Autodesk Inventor part; units mm, degrees
(part 2 of 2)
sketch "スケッチ4" plane through (0, 0, 0) normal (0, 0, 1) x (1, 0, 0)
  circle A0 centre (0, 0) radius 11.0288
  circle A1 centre (0, 0) radius 27.25
  circle A2 centre (0, 0) radius 22.25
  circle A3 centre (0, 0) radius 11.5288
  line L0 (-27.25, 0) -> (27.25, 0)
  line L1 (0, -27.25) -> (0, 27.25)
  line L2 (22.1994, 1.5) -> (11.2545, 2.5)
  line L3 (22.1994, -1.5) -> (11.2545, -2.5)
  line L4 (2.5, -11.2545) -> (1.5, -22.1994)
  line L5 (-2.5, -11.2545) -> (-1.5, -22.1994)
  line L6 (-22.1994, -1.5) -> (-11.2545, -2.5)
  line L7 (-11.2545, 2.5) -> (-22.1994, 1.5)
  line L8 (-1.5, 22.1994) -> (-2.5, 11.2545)
  line L9 (2.5, 11.2545) -> (1.5, 22.1994)
  point P0 (10.1524, 4.3085)
  point P1 (19.2887, 19.2486)
  dimension "d8" = 0.5
  dimension "d7" = 5
  dimension "d9" = 1.5
  dimension "d10" = 1.5
  dimension "d11" = 1.5
  dimension "d12" = 1.5
  dimension "d13" = 1.5
  dimension "d14" = 1.5
  dimension "d15" = 1.5
  dimension "d16" = 1.5
  dimension "d17" = 2.5
  dimension "d18" = 2.5
  dimension "d19" = 2.5
  dimension "d20" = 2.5
  dimension "d21" = 2.5
  dimension "d22" = 2.5
  dimension "d23" = 2.5
  dimension "d24" = 2.5
  constraints: 20 end point, 3 coincident, 3 point on circle, 2 midpoint, 1 centre point, 1 horizontal, 1 vertical, 23 other
  measures "d9" distance from line of L0 L3.start
  measures "d10" distance from line of L0 L2.start
  measures "d11" distance from line of L1 L4.end
  measures "d12" distance from line of L5.end L1
  measures "d13" distance from line of L0 L6.start
  measures "d14" distance from line of L0 L7.end
  measures "d15" distance from line of L1 L8.start
  measures "d16" distance from line of L1 L9.end
  measures "d17" distance from line of L0 L2.end
  measures "d18" distance from line of L3.end L0
  measures "d19" distance from line of L1 L4.start
  measures "d20" distance from line of L1 L5.start
  measures "d21" distance from line of L0 L6.end
  measures "d22" distance from line of L0 L7.start
  measures "d23" distance from line of L1 L8.end
  measures "d24" distance from line of L1 L9.start
extrude "押し出し4" cut sketch "スケッチ4" against normal through all contours A3 L9 A2 L2 | L3 A2 L4 A3 | A3 L7 A2 L8 | L5 A2 L6 A3
fillet "フィレット1" radius 4 16 edges at (1.5, 22.1994, -2) (-1.5, 22.1994, -2) (-2.5, 11.2545, -2) (2.5, 11.2545, -2) (11.2545, 2.5, -2) (22.1994, 1.5, -2) (22.1994, -1.5, -2) (11.2545, -2.5, -2) (1.5, -22.1994, -2) (2.5, -11.2545, -2) (-1.5, -22.1994, -2) (-2.5, -11.2545, -2) (-11.2545, -2.5, -2) (-22.1994, -1.5, -2) (-22.1994, 1.5, -2) (-11.2545, 2.5, -2)
sketch "スケッチ5" plane through (0, 0, 8) normal (0, 0, 1) x (1, 0, 0)
  arc A0 (-10.5551, -4.6371) -> (-4.6371, -10.5551) centre (0, 0) ccw projected
  arc A1 (-2.2625, -13.8534) -> (-4.6371, -10.5551) centre (-6.246, -14.2173) ccw projected
  line L0 (-2.2625, -13.8534) -> (-1.9858, -16.8822) projected
  arc A2 (-7.2775, -21.0262) -> (-1.9858, -16.8822) centre (-5.9692, -17.2462) ccw projected
  arc A3 (-21.0262, -7.2775) -> (-7.2775, -21.0262) centre (0, 0) ccw projected
  arc A4 (-16.8822, -1.9858) -> (-21.0262, -7.2775) centre (-17.2462, -5.9692) ccw projected
  line L1 (-16.8822, -1.9858) -> (-13.8534, -2.2625) projected
  arc A5 (-10.5551, -4.6371) -> (-13.8534, -2.2625) centre (-14.2173, -6.246) ccw projected
  line L2 (1.9858, -16.8822) -> (2.2625, -13.8534) projected
  arc A6 (4.6371, -10.5551) -> (2.2625, -13.8534) centre (6.246, -14.2173) ccw projected
  arc A7 (4.6371, -10.5551) -> (10.5551, -4.6371) centre (0, 0) ccw projected
  arc A8 (13.8534, -2.2625) -> (10.5551, -4.6371) centre (14.2173, -6.246) ccw projected
  line L3 (13.8534, -2.2625) -> (16.8822, -1.9858) projected
  arc A9 (21.0262, -7.2775) -> (16.8822, -1.9858) centre (17.2462, -5.9692) ccw projected
  arc A10 (7.2775, -21.0262) -> (21.0262, -7.2775) centre (0, 0) ccw projected
  arc A11 (1.9858, -16.8822) -> (7.2775, -21.0262) centre (5.9692, -17.2462) ccw projected
  line L4 (-1.9858, 16.8822) -> (-2.2625, 13.8534) projected
  arc A12 (-4.6371, 10.5551) -> (-2.2625, 13.8534) centre (-6.246, 14.2173) ccw projected
  arc A13 (-4.6371, 10.5551) -> (-10.5551, 4.6371) centre (0, 0) ccw projected
  arc A14 (-13.8534, 2.2625) -> (-10.5551, 4.6371) centre (-14.2173, 6.246) ccw projected
  line L5 (-13.8534, 2.2625) -> (-16.8822, 1.9858) projected
  arc A15 (-21.0262, 7.2775) -> (-16.8822, 1.9858) centre (-17.2462, 5.9692) ccw projected
  arc A16 (-7.2775, 21.0262) -> (-21.0262, 7.2775) centre (0, 0) ccw projected
  arc A17 (-1.9858, 16.8822) -> (-7.2775, 21.0262) centre (-5.9692, 17.2462) ccw projected
  arc A18 (21.0262, 7.2775) -> (7.2775, 21.0262) centre (0, 0) ccw projected
  arc A19 (16.8822, 1.9858) -> (21.0262, 7.2775) centre (17.2462, 5.9692) ccw projected
  line L6 (16.8822, 1.9858) -> (13.8534, 2.2625) projected
  arc A20 (10.5551, 4.6371) -> (13.8534, 2.2625) centre (14.2173, 6.246) ccw projected
  arc A21 (10.5551, 4.6371) -> (4.6371, 10.5551) centre (0, 0) ccw projected
  arc A22 (2.2625, 13.8534) -> (4.6371, 10.5551) centre (6.246, 14.2173) ccw projected
  line L7 (2.2625, 13.8534) -> (1.9858, 16.8822) projected
  arc A23 (7.2775, 21.0262) -> (1.9858, 16.8822) centre (5.9692, 17.2462) ccw projected
  arc A24 (-14.6125, 23.0008) -> (-14.9971, 23.3759) centre (-19.1364, 18.7478) ccw projected
  arc A25 (-14.9971, 23.3759) -> (-15.5935, 23.8634) centre (-20.7203, 16.9823) ccw projected
  arc A26 (-15.5935, 23.8634) -> (-16.4862, 24.4634) centre (-22.2157, 14.9751) ccw projected
  arc A27 (-16.4862, 24.4634) -> (-17.1295, 24.0173) centre (0, 0) ccw projected
  arc A28 (-17.1295, 24.0173) -> (-16.8828, 22.9783) centre (-6.2347, 26.0561) ccw projected
  arc A29 (-16.8828, 22.9783) -> (-16.6333, 22.2415) centre (-8.6388, 25.3594) ccw projected
  arc A30 (-16.6333, 22.2415) -> (-16.4168, 21.7498) centre (-10.8476, 24.4952) ccw projected
  arc A31 (-16.4168, 21.7498) -> (-17.0541, 21.2537) centre (0, 0) ccw projected
  arc A32 (-17.0541, 21.2537) -> (-17.4777, 21.5843) centre (-21.0827, 16.5289) ccw projected
  arc A33 (-17.4777, 21.5843) -> (-18.1241, 22.0031) centre (-22.4627, 14.5998) ccw projected
  arc A34 (-18.1241, 22.0031) -> (-19.0773, 22.5013) centre (-23.7282, 12.4403) ccw projected
  arc A35 (-19.0773, 22.5013) -> (-19.6677, 21.9871) centre (0, 0) ccw projected
  arc A36 (-19.6677, 21.9871) -> (-19.3081, 20.9816) centre (-9.0632, 25.2121) ccw projected
  arc A37 (-19.3081, 20.9816) -> (-18.9791, 20.2767) centre (-11.3761, 24.2551) ccw projected
  arc A38 (-18.9791, 20.2767) -> (-18.7098, 19.8118) centre (-13.4764, 23.1532) ccw projected
  arc A39 (-18.7098, 19.8118) -> (-19.2887, 19.2486) centre (0, 0) ccw projected
  arc A40 (-19.2887, 19.2486) -> (-19.746, 19.5306) centre (-22.773, 14.1093) ccw projected
  arc A41 (-19.746, 19.5306) -> (-20.4346, 19.8758) centre (-23.9325, 12.0401) ccw projected
  arc A42 (-20.4346, 19.8758) -> (-21.4368, 20.2661) centre (-24.9528, 9.7545) ccw projected
  arc A43 (-21.4368, 20.2661) -> (-21.9671, 19.69) centre (0, 0) ccw projected
  arc A44 (-21.9671, 19.69) -> (-21.4954, 18.7235) centre (-11.7818, 24.062) ccw projected
  arc A45 (-21.4954, 18.7235) -> (-21.0945, 18.0658) centre (-13.9753, 22.8564) ccw projected
  arc A46 (-21.0945, 18.0658) -> (-20.7757, 17.6333) centre (-15.9417, 21.5301) ccw projected
  arc A47 (-20.7757, 17.6333) -> (-21.2891, 17.0099) centre (0, 0) ccw projected
  arc A48 (-21.2891, 17.0099) -> (-21.7747, 17.2398) centre (-24.187, 11.5184) ccw projected
  arc A49 (-21.7747, 17.2398) -> (-22.4971, 17.5072) centre (-25.1117, 9.3343) ccw projected
  arc A50 (-22.4971, 17.5072) -> (-23.5361, 17.7848) centre (-25.8744, 6.9503) ccw projected
  arc A51 (-23.5361, 17.7848) -> (-23.9998, 17.154) centre (0, 0) ccw projected
  arc A52 (-23.9998, 17.154) -> (-23.4247, 16.2452) centre (-14.3573, 22.6199) ccw projected
  arc A53 (-23.4247, 16.2452) -> (-22.9538, 15.6355) centre (-16.4049, 21.1803) ccw projected
  arc A54 (-22.9538, 15.6355) -> (-22.5894, 15.2408) centre (-18.2134, 19.6457) ccw projected
  arc A55 (-22.5894, 15.2408) -> (-23.0312, 14.5646) centre (0, 0) ccw projected
  arc A56 (-23.0312, 14.5646) -> (-23.5391, 14.7398) centre (-25.3073, 8.7878) ccw projected
  arc A57 (-23.5391, 14.7398) -> (-24.294, 14.9276) centre (-25.9861, 6.5151) ccw projected
  arc A58 (-24.294, 14.9276) -> (-25.3498, 15.0877) centre (-26.4819, 4.0617) ccw projected
  arc A59 (-25.3498, 15.0877) -> (-25.7412, 14.4097) centre (0, 0) ccw projected
  arc A60 (-25.7412, 14.4097) -> (-25.0747, 13.5754) centre (-16.7585, 20.9032) ccw projected
  arc A61 (-25.0747, 13.5754) -> (-24.5345, 13.0155) centre (-18.6353, 19.2471) ccw projected
  arc A62 (-24.5345, 13.0155) -> (-24.1289, 12.6632) centre (-20.2641, 17.5229) ccw projected
  arc A63 (-24.1289, 12.6632) -> (-24.4936, 11.9426) centre (0, 0) ccw projected
  arc A64 (-24.4936, 11.9426) -> (-25.0177, 12.0608) centre (-26.1204, 5.9504) ccw projected
  arc A65 (-25.0177, 12.0608) -> (-25.7887, 12.1645) centre (-26.5451, 3.6169) ccw projected
  arc A66 (-25.7887, 12.1645) -> (-26.8557, 12.2075) centre (-26.768, 1.1238) ccw projected
  arc A67 (-26.8557, 12.2075) -> (-27.1702, 11.4905) centre (0, 0) ccw projected
  arc A68 (-27.1702, 11.4905) -> (-26.4159, 10.7346) centre (-18.9563, 18.9327) ccw projected
  arc A69 (-26.4159, 10.7346) -> (-25.8175, 10.2375) centre (-20.6396, 17.0802) ccw projected
  arc A70 (-25.8175, 10.2375) -> (-25.3755, 9.932) centre (-22.0687, 15.1873) ccw projected
  arc A71 (-25.3755, 9.932) -> (-25.6587, 9.1756) centre (0, 0) ccw projected
  arc A72 (-25.6587, 9.1756) -> (-26.1926, 9.2355) centre (-26.6165, 3.0408) ccw projected
  arc A73 (-26.1926, 9.2355) -> (-26.9703, 9.2537) centre (-26.7819, 0.6748) ccw projected
  arc A74 (-26.9703, 9.2537) -> (-28.0356, 9.179) centre (-26.7292, -1.8277) ccw projected
  arc A75 (-28.0356, 9.179) -> (-28.2693, 8.4318) centre (0, 0) ccw projected
  arc A76 (-28.2693, 8.4318) -> (-27.4364, 7.7635) centre (-20.924, 16.7325) ccw projected
  arc A77 (-27.4364, 7.7635) -> (-26.787, 7.3353) centre (-22.3933, 14.7061) ccw projected
  arc A78 (-26.787, 7.3353) -> (-26.3141, 7.0802) centre (-23.6055, 12.6674) ccw projected
  arc A79 (-26.3141, 7.0802) -> (-26.5124, 6.2973) centre (0, 0) ccw projected
  arc A80 (-26.5124, 6.2973) -> (-27.0496, 6.298) centre (-26.7894, 0.0943) ccw projected
  arc A81 (-27.0496, 6.298) -> (-27.8246, 6.2305) centre (-26.6936, -2.2756) ccw projected
  arc A82 (-27.8246, 6.2305) -> (-28.8752, 6.0392) centre (-26.3659, -4.757) ccw projected
  arc A83 (-28.8752, 6.0392) -> (-29.0253, 5.2708) centre (0, 0) ccw projected
  arc A84 (-29.0253, 5.2708) -> (-28.124, 4.6981) centre (-22.6377, 14.3291) ccw projected
  arc A85 (-28.124, 4.6981) -> (-27.4313, 4.344) centre (-23.8751, 12.1534) ccw projected
  arc A86 (-27.4313, 4.344) -> (-26.9333, 4.1425) centre (-24.8558, 9.9937) ccw projected
  arc A87 (-26.9333, 4.1425) -> (-27.0442, 3.3425) centre (0, 0) ccw projected
  arc A88 (-27.0442, 3.3425) -> (-27.5783, 3.2841) centre (-26.6372, -2.8533) ccw projected
  arc A89 (-27.5783, 3.2841) -> (-28.3412, 3.1318) centre (-26.2813, -5.1983) ccw projected
  arc A90 (-28.3412, 3.1318) -> (-29.3643, 2.826) centre (-25.6826, -7.6286) ccw projected
  arc A91 (-29.3643, 2.826) -> (-29.429, 2.0458) centre (0, 0) ccw projected
  arc A92 (-29.429, 2.0458) -> (-28.4631, 1.5727) centre (-24.0767, 11.7518) ccw projected
  arc A93 (-28.4631, 1.5727) -> (-27.7427, 1.2999) centre (-25.0672, 9.4531) ccw projected
  arc A94 (-27.7427, 1.2999) -> (-27.2255, 1.1544) centre (-25.8043, 7.1987) ccw projected
  arc A95 (-27.2255, 1.1544) -> (-27.2478, 0.3471) centre (0, 0) ccw projected
  arc A96 (-27.2478, 0.3471) -> (-27.7722, 0.2303) centre (-26.1617, -5.7663) ccw projected
  arc A97 (-27.7722, 0.2303) -> (-28.5137, -0.005) centre (-25.5499, -8.0579) ccw projected
  arc A98 (-28.5137, -0.005) -> (-29.497, -0.4215) centre (-24.6875, -10.4076) ccw projected
  arc A99 (-29.497, -0.4215) -> (-29.4754, -1.2041) centre (0, 0) ccw projected
  arc A100 (-29.4754, -1.2041) -> (-28.4706, -1.5658) centre (-25.2233, 9.0318) ccw projected
  arc A101 (-28.4706, -1.5658) -> (-27.7173, -1.7599) centre (-25.955, 6.6382) ccw projected
  arc A102 (-27.7173, -1.7599) -> (-27.1873, -1.8476) centre (-26.4396, 4.3163) ccw projected
  arc A103 (-27.1873, -1.8476) -> (-27.1206, -2.6525) centre (0, 0) ccw projected
  arc A104 (-27.1206, -2.6525) -> (-27.629, -2.8262) centre (-25.3685, -8.6093) ccw projected
  arc A105 (-27.629, -2.8262) -> (-28.3401, -3.1417) centre (-24.5084, -10.8197) ccw projected
  arc A106 (-28.3401, -3.1417) -> (-29.2716, -3.6638) centre (-23.3927, -13.0603) ccw projected
  arc A107 (-29.2716, -3.6638) -> (-29.1641, -4.4393) centre (0, 0) ccw projected
  arc A108 (-29.1641, -4.4393) -> (-28.1256, -4.6883) centre (-26.0638, 6.2023) ccw projected
  arc A109 (-28.1256, -4.6883) -> (-27.3555, -4.7983) centre (-26.5277, 3.7426) ccw projected
  arc A110 (-27.3555, -4.7983) -> (-26.819, -4.8272) centre (-26.754, 1.3816) ccw projected
  arc A111 (-26.819, -4.8272) -> (-26.6642, -5.6199) centre (0, 0) ccw projected
  arc A112 (-26.6642, -5.6199) -> (-27.1504, -5.8485) centre (-24.2675, -11.3478) ccw projected
  arc A113 (-27.1504, -5.8485) -> (-27.8224, -6.2403) centre (-23.1694, -13.4501) ccw projected
  arc A114 (-27.8224, -6.2403) -> (-28.6909, -6.8617) centre (-21.814, -15.5544) ccw projected
  arc A115 (-28.6909, -6.8617) -> (-28.4987, -7.6207) centre (0, 0) ccw projected
  arc A116 (-28.4987, -7.6207) -> (-27.4392, -7.7539) centre (-26.5879, 3.2974) ccw projected
  arc A117 (-27.4392, -7.7539) -> (-26.6616, -7.7786) centre (-26.7784, 0.8016) ccw projected
  arc A118 (-26.6616, -7.7786) -> (-26.1252, -7.7482) centre (-26.7436, -1.57) ccw projected
  arc A119 (-26.1252, -7.7482) -> (-25.8841, -8.519) centre (0, 0) ccw projected
  arc A120 (-25.8841, -8.519) -> (-26.3422, -8.7998) centre (-22.8719, -13.9485) ccw projected
  arc A121 (-26.3422, -8.7998) -> (-26.9671, -9.2631) centre (-21.5491, -15.9173) ccw projected
  arc A122 (-26.9671, -9.2631) -> (-27.7619, -9.9763) centre (-19.9705, -17.8597) ccw projected
  arc A123 (-27.7619, -9.9763) -> (-27.4874, -10.7095) centre (0, 0) ccw projected
  arc A124 (-27.4874, -10.7095) -> (-26.4196, -10.7253) centre (-26.7893, 0.3525) ccw projected
  arc A125 (-26.4196, -10.7253) -> (-25.6441, -10.6643) centre (-26.7041, -2.1491) ccw projected
  arc A126 (-25.6441, -10.6643) -> (-25.1143, -10.5752) centre (-26.4085, -4.5025) ccw projected
  arc A127 (-25.1143, -10.5752) -> (-24.7899, -11.3148) centre (0, 0) ccw projected
  arc A128 (-24.7899, -11.3148) -> (-25.2143, -11.6442) centre (-21.1986, -16.38) ccw projected
  arc A129 (-25.2143, -11.6442) -> (-25.7844, -12.1735) centre (-19.6673, -18.1913) ccw projected
  arc A130 (-25.7844, -12.1735) -> (-26.4959, -12.9698) centre (-17.8846, -19.9482) ccw projected
  arc A131 (-26.4959, -12.9698) -> (-26.1424, -13.6683) centre (0, 0) ccw projected
  arc A132 (-26.1424, -13.6683) -> (-25.0794, -13.5666) centre (-26.6655, -2.5967) ccw projected
  arc A133 (-25.0794, -13.5666) -> (-24.3153, -13.4207) centre (-26.3056, -5.0737) ccw projected
  arc A134 (-24.3153, -13.4207) -> (-23.7985, -13.2738) centre (-25.7529, -7.3803) ccw projected
  arc A135 (-23.7985, -13.2738) -> (-23.3947, -13.9732) centre (0, 0) ccw projected
  arc A136 (-23.3947, -13.9732) -> (-23.7803, -14.3473) centre (-19.268, -18.6126) ccw projected
  arc A137 (-23.7803, -14.3473) -> (-24.2887, -14.9361) centre (-17.5468, -20.2445) ccw projected
  arc A138 (-24.2887, -14.9361) -> (-24.9083, -15.8058) centre (-15.5815, -21.7946) ccw projected
  arc A139 (-24.9083, -15.8058) -> (-24.4801, -16.4613) centre (0, 0) ccw projected
  arc A140 (-24.4801, -16.4613) -> (-23.4347, -16.2432) centre (-26.218, -5.5144) ccw projected
  arc A141 (-23.4347, -16.2432) -> (-22.6913, -16.0141) centre (-25.5878, -7.9368) ccw projected
  arc A142 (-22.6913, -16.0141) -> (-22.1938, -15.8113) centre (-24.7848, -10.1685) ccw projected
  arc A143 (-22.1938, -15.8113) -> (-21.7155, -16.462) centre (0, 0) ccw projected
  arc A144 (-21.7155, -16.462) -> (-22.0576, -16.8763) centre (-17.1035, -20.6192) ccw projected
  arc A145 (-22.0576, -16.8763) -> (-22.4982, -17.5174) centre (-15.2132, -22.0519) ccw projected
  arc A146 (-22.4982, -17.5174) -> (-23.0184, -18.45) centre (-13.0894, -23.3764) ccw projected
  arc A147 (-23.0184, -18.45) -> (-22.5207, -19.0544) centre (0, 0) ccw projected
  arc A148 (-22.5207, -19.0544) -> (-21.5056, -18.7227) centre (-25.4522, -8.3651) ccw projected
  arc A149 (-21.5056, -18.7227) -> (-20.7919, -18.4131) centre (-24.5594, -10.7034) ccw projected
  arc A150 (-20.7919, -18.4131) -> (-20.3198, -18.1568) centre (-23.5157, -12.8333) ccw projected
  arc A151 (-20.3198, -18.1568) -> (-19.7728, -18.751) centre (0, 0) ccw projected
  arc A152 (-19.7728, -18.751) -> (-20.0672, -19.2004) centre (-14.7314, -22.3756) ccw projected
  arc A153 (-20.0672, -19.2004) -> (-20.4346, -19.8861) centre (-12.695, -23.5916) ccw projected
  arc A154 (-20.4346, -19.8861) -> (-20.849, -20.8703) centre (-10.4383, -24.6745) ccw projected
  arc A155 (-20.849, -20.8703) -> (-20.2879, -21.4162) centre (0, 0) ccw projected
  arc A156 (-20.2879, -21.4162) -> (-19.3155, -20.9748) centre (-24.3775, -11.1143) ccw projected
  arc A157 (-19.3155, -20.9748) -> (-18.6401, -20.5887) centre (-23.2328, -13.3402) ccw projected
  arc A158 (-18.6401, -20.5887) -> (-18.1991, -20.2819) centre (-21.9612, -15.3424) ccw projected
  arc A159 (-18.1991, -20.2819) -> (-17.59, -20.8124) centre (0, 0) ccw projected
  arc A160 (-17.59, -20.8124) -> (-17.8332, -21.2914) centre (-12.1805, -23.8604) ccw projected
  arc A161 (-17.8332, -21.2914) -> (-18.123, -22.0133) centre (-10.0227, -24.845) ccw projected
  arc A162 (-18.123, -22.0133) -> (-18.4266, -23.0372) centre (-7.6606, -25.6731) ccw projected
  arc A163 (-18.4266, -23.0372) -> (-17.8088, -23.518) centre (0, 0) ccw projected
  arc A164 (-17.8088, -23.518) -> (-16.8908, -22.9724) centre (-23.0069, -13.7285) ccw projected
  arc A165 (-16.8908, -22.9724) -> (-16.2621, -22.5143) centre (-21.6243, -15.8151) ccw projected
  arc A166 (-16.2621, -22.5143) -> (-15.8574, -22.1609) centre (-20.1401, -17.6652) ccw projected
  arc A167 (-15.8574, -22.1609) -> (-15.1937, -22.6211) centre (0, 0) ccw projected
  arc A168 (-15.1937, -22.6211) -> (-15.3828, -23.124) centre (-9.4817, -25.0555) ccw projected
  arc A169 (-15.3828, -23.124) -> (-15.5913, -23.8734) centre (-7.2287, -25.7968) ccw projected
  arc A170 (-15.5913, -23.8734) -> (-15.7805, -24.9244) centre (-4.7899, -26.36) ccw projected
  arc A171 (-15.7805, -24.9244) -> (-15.1135, -25.3344) centre (0, 0) ccw projected
  arc A172 (-15.1135, -25.3344) -> (-14.2612, -24.6911) centre (-21.357, -16.1762) ccw projected
  arc A173 (-14.2612, -24.6911) -> (-13.6866, -24.1666) centre (-19.7533, -18.0979) ccw projected
  arc A174 (-13.6866, -24.1666) -> (-13.3233, -23.7708) centre (-18.0746, -19.7735) ccw projected
  arc A175 (-13.3233, -23.7708) -> (-12.613, -24.1552) centre (0, 0) ccw projected
  arc A176 (-12.613, -24.1552) -> (-12.7456, -24.6759) centre (-6.6679, -25.9465) ccw projected
  arc A177 (-12.7456, -24.6759) -> (-12.8704, -25.4437) centre (-4.347, -26.4354) ccw projected
  arc A178 (-12.8704, -25.4437) -> (-12.9428, -26.5091) centre (-1.861, -26.7269) ccw projected
  arc A179 (-12.9428, -26.5091) -> (-12.2348, -26.8433) centre (0, 0) ccw projected
  arc A180 (-12.2348, -26.8433) -> (-11.4584, -26.1101) centre (-19.4479, -18.4274) ccw projected
  arc A181 (-11.4584, -26.1101) -> (-10.945, -25.5256) centre (-17.6425, -20.1611) ccw projected
  arc A182 (-10.945, -25.5256) -> (-10.6274, -25.0922) centre (-15.7896, -21.6419) ccw projected
  arc A183 (-10.6274, -25.0922) -> (-9.8792, -25.3962) centre (0, 0) ccw projected
  arc A184 (-9.8792, -25.3962) -> (-9.9537, -25.9282) centre (-3.7731, -26.5226) ccw projected
  arc A185 (-9.9537, -25.9282) -> (-9.9933, -26.7051) centre (-1.4125, -26.7532) ccw projected
  arc A186 (-9.9933, -26.7051) -> (-9.948, -27.772) centre (1.0905, -26.7694) ccw projected
  arc A187 (-9.948, -27.772) -> (-9.2075, -28.0263) centre (0, 0) ccw projected
  arc A188 (-9.2075, -28.0263) -> (-8.5165, -27.2121) centre (-17.3027, -20.455) ccw projected
  arc A189 (-8.5165, -27.2121) -> (-8.0706, -26.5747) centre (-15.3175, -21.9796) ccw projected
  arc A190 (-8.0706, -26.5747) -> (-7.8026, -26.109) centre (-13.313, -23.2475) ccw projected
  arc A191 (-7.8026, -26.109) -> (-7.0254, -26.3288) centre (0, 0) ccw projected
  arc A192 (-7.0254, -26.3288) -> (-7.041, -26.8658) centre (-0.8325, -26.7767) ccw projected
  arc A193 (-7.041, -26.8658) -> (-6.9957, -27.6348) centre (1.5392, -26.7462) ccw projected
  arc A194 (-6.9957, -27.6348) -> (-6.8325, -28.6979) centre (4.0287, -26.487) ccw projected
  arc A195 (-6.8325, -28.6979) -> (-6.0685, -28.8691) centre (0, 0) ccw projected
  arc A196 (-6.0685, -28.8691) -> (-5.4713, -27.9838) centre (-14.9474, -22.2343) ccw projected
  arc A197 (-5.4713, -27.9838) -> (-5.0982, -27.3012) centre (-12.8066, -23.5312) ccw projected
  arc A198 (-5.0982, -27.3012) -> (-4.883, -26.8089) centre (-10.6748, -24.571) ccw projected
  arc A199 (-4.883, -26.8089) -> (-4.0864, -26.9419) centre (0, 0) ccw projected
  arc A200 (-4.0864, -26.9419) -> (-4.0428, -27.4773) centre (2.1182, -26.7057) ccw projected
  arc A201 (-4.0428, -27.4773) -> (-3.9115, -28.2441) centre (4.4721, -26.4145) ccw projected
  arc A202 (-3.9115, -28.2441) -> (-3.634, -29.2753) centre (6.9181, -25.883) ccw projected
  arc A203 (-3.634, -29.2753) -> (-2.8559, -29.3614) centre (0, 0) ccw projected
  arc A204 (-2.8559, -29.3614) -> (-2.3596, -28.4159) centre (-12.4108, -23.7437) ccw projected
  arc A205 (-2.3596, -28.4159) -> (-2.0639, -27.6964) centre (-10.1402, -24.7972) ccw projected
  arc A206 (-2.0639, -27.6964) -> (-1.9042, -27.1834) centre (-7.907, -25.5961) ccw projected
  arc A207 (-1.9042, -27.1834) -> (-1.0978, -27.2279) centre (0, 0) ccw projected
  arc A208 (-1.0978, -27.2279) -> (-0.9955, -27.7553) centre (5.0432, -26.3106) ccw projected
  arc A209 (-0.9955, -27.7553) -> (-0.7807, -28.503) centre (7.3508, -25.7622) ccw projected
  arc A210 (-0.7807, -28.503) -> (-0.3915, -29.4974) centre (9.7234, -24.9649) ccw projected
  arc A211 (-0.3915, -29.4974) -> (0.3915, -29.4974) centre (0, 0) ccw projected
  arc A212 (0.3915, -29.4974) -> (0.7807, -28.503) centre (-9.7234, -24.9649) ccw projected
  arc A213 (0.7807, -28.503) -> (0.9955, -27.7553) centre (-7.3508, -25.7622) ccw projected
  arc A214 (0.9955, -27.7553) -> (1.0978, -27.2279) centre (-5.0432, -26.3106) ccw projected
  arc A215 (1.0978, -27.2279) -> (1.9042, -27.1834) centre (0, 0) ccw projected
  arc A216 (1.9042, -27.1834) -> (2.0639, -27.6964) centre (7.907, -25.5961) ccw projected
  arc A217 (2.0639, -27.6964) -> (2.3596, -28.4159) centre (10.1402, -24.7972) ccw projected
  arc A218 (2.3596, -28.4159) -> (2.8559, -29.3614) centre (12.4108, -23.7437) ccw projected
  arc A219 (2.8559, -29.3614) -> (3.634, -29.2753) centre (0, 0) ccw projected
  arc A220 (3.634, -29.2753) -> (3.9115, -28.2441) centre (-6.9181, -25.883) ccw projected
  arc A221 (3.9115, -28.2441) -> (4.0428, -27.4773) centre (-4.4721, -26.4145) ccw projected
  arc A222 (4.0428, -27.4773) -> (4.0864, -26.9419) centre (-2.1182, -26.7057) ccw projected
  arc A223 (4.0864, -26.9419) -> (4.883, -26.8089) centre (0, 0) ccw projected
  arc A224 (4.883, -26.8089) -> (5.0982, -27.3012) centre (10.6748, -24.571) ccw projected
  arc A225 (5.0982, -27.3012) -> (5.4713, -27.9838) centre (12.8066, -23.5312) ccw projected
  arc A226 (5.4713, -27.9838) -> (6.0685, -28.8691) centre (14.9474, -22.2343) ccw projected
  arc A227 (6.0685, -28.8691) -> (6.8325, -28.6979) centre (0, 0) ccw projected
  arc A228 (6.8325, -28.6979) -> (6.9949, -27.6424) centre (-4.0287, -26.487) ccw projected
  arc A229 (6.9949, -27.6424) -> (7.041, -26.8658) centre (-1.5392, -26.7462) ccw projected
  arc A230 (7.041, -26.8658) -> (7.0254, -26.3288) centre (0.8325, -26.7767) ccw projected
  arc A231 (7.0254, -26.3288) -> (7.8026, -26.109) centre (0, 0) ccw projected
  arc A232 (7.8026, -26.109) -> (8.0706, -26.5747) centre (13.313, -23.2475) ccw projected
  arc A233 (8.0706, -26.5747) -> (8.5165, -27.2121) centre (15.3175, -21.9796) ccw projected
  arc A234 (8.5165, -27.2121) -> (9.2075, -28.0263) centre (17.3027, -20.455) ccw projected
  arc A235 (9.2075, -28.0263) -> (9.948, -27.772) centre (0, 0) ccw projected
  arc A236 (9.948, -27.772) -> (9.9933, -26.7051) centre (-1.0905, -26.7694) ccw projected
  arc A237 (9.9933, -26.7051) -> (9.9537, -25.9282) centre (1.4125, -26.7532) ccw projected
  arc A238 (9.9537, -25.9282) -> (9.8792, -25.3962) centre (3.7731, -26.5226) ccw projected
  arc A239 (9.8792, -25.3962) -> (10.6274, -25.0922) centre (0, 0) ccw projected
  arc A240 (10.6274, -25.0922) -> (10.945, -25.5256) centre (15.7896, -21.6419) ccw projected
  arc A241 (10.945, -25.5256) -> (11.4584, -26.1101) centre (17.6425, -20.1611) ccw projected
  arc A242 (11.4584, -26.1101) -> (12.2348, -26.8433) centre (19.4479, -18.4274) ccw projected
  arc A243 (12.2348, -26.8433) -> (12.9428, -26.5091) centre (0, 0) ccw projected
  arc A244 (12.9428, -26.5091) -> (12.8704, -25.4437) centre (1.861, -26.7269) ccw projected
  arc A245 (12.8704, -25.4437) -> (12.7456, -24.6759) centre (4.347, -26.4354) ccw projected
  arc A246 (12.7456, -24.6759) -> (12.613, -24.1552) centre (6.6679, -25.9465) ccw projected
  arc A247 (12.613, -24.1552) -> (13.3233, -23.7708) centre (0, 0) ccw projected
  arc A248 (13.3233, -23.7708) -> (13.6866, -24.1666) centre (18.0746, -19.7735) ccw projected
  arc A249 (13.6866, -24.1666) -> (14.2612, -24.6911) centre (19.7533, -18.0979) ccw projected
  arc A250 (14.2612, -24.6911) -> (15.1135, -25.3344) centre (21.357, -16.1762) ccw projected
  arc A251 (15.1135, -25.3344) -> (15.7805, -24.9244) centre (0, 0) ccw projected
  arc A252 (15.7805, -24.9244) -> (15.5913, -23.8734) centre (4.7899, -26.36) ccw projected
  arc A253 (15.5913, -23.8734) -> (15.3828, -23.124) centre (7.2287, -25.7968) ccw projected
  arc A254 (15.3828, -23.124) -> (15.1937, -22.6211) centre (9.4817, -25.0555) ccw projected
  arc A255 (15.1937, -22.6211) -> (15.8574, -22.1609) centre (0, 0) ccw projected
  arc A256 (15.8574, -22.1609) -> (16.2621, -22.5143) centre (20.1401, -17.6652) ccw projected
  arc A257 (16.2621, -22.5143) -> (16.8908, -22.9724) centre (21.6243, -15.8151) ccw projected
  arc A258 (16.8908, -22.9724) -> (17.8088, -23.518) centre (23.0069, -13.7285) ccw projected
  arc A259 (17.8088, -23.518) -> (18.4266, -23.0372) centre (0, 0) ccw projected
  arc A260 (18.4266, -23.0372) -> (18.123, -22.0134) centre (7.6606, -25.6731) ccw projected
  arc A261 (18.123, -22.0134) -> (17.8332, -21.2914) centre (10.0227, -24.845) ccw projected
  arc A262 (17.8332, -21.2914) -> (17.59, -20.8124) centre (12.1805, -23.8604) ccw projected
  arc A263 (17.59, -20.8124) -> (18.1991, -20.2819) centre (0, 0) ccw projected
  arc A264 (18.1991, -20.2819) -> (18.6401, -20.5887) centre (21.9612, -15.3424) ccw projected
  arc A265 (18.6401, -20.5887) -> (19.3155, -20.9748) centre (23.2328, -13.3402) ccw projected
  arc A266 (19.3155, -20.9748) -> (20.2879, -21.4162) centre (24.3775, -11.1143) ccw projected
  arc A267 (20.2879, -21.4162) -> (20.849, -20.8703) centre (0, 0) ccw projected
  arc A268 (20.849, -20.8703) -> (20.4313, -19.8792) centre (10.4383, -24.6745) ccw projected
  arc A269 (20.4313, -19.8792) -> (20.0672, -19.2004) centre (12.695, -23.5916) ccw projected
  arc A270 (20.0672, -19.2004) -> (19.7728, -18.751) centre (14.7314, -22.3756) ccw projected
  arc A271 (19.7728, -18.751) -> (20.3198, -18.1568) centre (0, 0) ccw projected
  arc A272 (20.3198, -18.1568) -> (20.7919, -18.4131) centre (23.5157, -12.8333) ccw projected
  arc A273 (20.7919, -18.4131) -> (21.5056, -18.7227) centre (24.5594, -10.7034) ccw projected
  arc A274 (21.5056, -18.7227) -> (22.5207, -19.0544) centre (25.4522, -8.3651) ccw projected
  arc A275 (22.5207, -19.0544) -> (23.0184, -18.45) centre (0, 0) ccw projected
  arc A276 (23.0184, -18.45) -> (22.4982, -17.5174) centre (13.0894, -23.3764) ccw projected
  arc A277 (22.4982, -17.5174) -> (22.0576, -16.8763) centre (15.2132, -22.0519) ccw projected
  arc A278 (22.0576, -16.8763) -> (21.7155, -16.462) centre (17.1035, -20.6192) ccw projected
  arc A279 (21.7155, -16.462) -> (22.1938, -15.8113) centre (0, 0) ccw projected
  arc A280 (22.1938, -15.8113) -> (22.6913, -16.0141) centre (24.7848, -10.1685) ccw projected
  arc A281 (22.6913, -16.0141) -> (23.4347, -16.2432) centre (25.5878, -7.9368) ccw projected
  arc A282 (23.4347, -16.2432) -> (24.4801, -16.4613) centre (26.218, -5.5144) ccw projected
  arc A283 (24.4801, -16.4613) -> (24.9083, -15.8058) centre (0, 0) ccw projected
  arc A284 (24.9083, -15.8058) -> (24.2887, -14.9361) centre (15.5815, -21.7946) ccw projected
  arc A285 (24.2887, -14.9361) -> (23.7803, -14.3473) centre (17.5468, -20.2445) ccw projected
  arc A286 (23.7803, -14.3473) -> (23.3947, -13.9732) centre (19.268, -18.6126) ccw projected
  arc A287 (23.3947, -13.9732) -> (23.7985, -13.2738) centre (0, 0) ccw projected
  arc A288 (23.7985, -13.2738) -> (24.3153, -13.4207) centre (25.7529, -7.3803) ccw projected
  arc A289 (24.3153, -13.4207) -> (25.0794, -13.5666) centre (26.3056, -5.0737) ccw projected
  arc A290 (25.0794, -13.5666) -> (26.1424, -13.6683) centre (26.6655, -2.5967) ccw projected
  arc A291 (26.1424, -13.6683) -> (26.4959, -12.9698) centre (0, 0) ccw projected
  arc A292 (26.4959, -12.9698) -> (25.7844, -12.1735) centre (17.8846, -19.9482) ccw projected
  arc A293 (25.7844, -12.1735) -> (25.2143, -11.6442) centre (19.6673, -18.1913) ccw projected
  arc A294 (25.2143, -11.6442) -> (24.7899, -11.3148) centre (21.1986, -16.38) ccw projected
  arc A295 (24.7899, -11.3148) -> (25.1143, -10.5752) centre (0, 0) ccw projected
  arc A296 (25.1143, -10.5752) -> (25.6441, -10.6643) centre (26.4085, -4.5025) ccw projected
  arc A297 (25.6441, -10.6643) -> (26.4196, -10.7253) centre (26.7041, -2.1491) ccw projected
  arc A298 (26.4196, -10.7253) -> (27.4874, -10.7095) centre (26.7893, 0.3525) ccw projected
  arc A299 (27.4874, -10.7095) -> (27.7619, -9.9763) centre (0, 0) ccw projected
  arc A300 (27.7619, -9.9763) -> (26.9671, -9.2631) centre (19.9705, -17.8597) ccw projected
  arc A301 (26.9671, -9.2631) -> (26.3422, -8.7998) centre (21.5491, -15.9173) ccw projected
  arc A302 (26.3422, -8.7998) -> (25.8841, -8.519) centre (22.8719, -13.9485) ccw projected
  arc A303 (25.8841, -8.519) -> (26.1252, -7.7482) centre (0, 0) ccw projected
  arc A304 (26.1252, -7.7482) -> (26.6616, -7.7786) centre (26.7436, -1.57) ccw projected
  arc A305 (26.6616, -7.7786) -> (27.4392, -7.7539) centre (26.7784, 0.8016) ccw projected
  arc A306 (27.4392, -7.7539) -> (28.4987, -7.6207) centre (26.5879, 3.2974) ccw projected
  arc A307 (28.4987, -7.6207) -> (28.6909, -6.8617) centre (0, 0) ccw projected
  arc A308 (28.6909, -6.8617) -> (27.8224, -6.2403) centre (21.814, -15.5544) ccw projected
  arc A309 (27.8224, -6.2403) -> (27.1504, -5.8485) centre (23.1694, -13.4501) ccw projected
  arc A310 (27.1504, -5.8485) -> (26.6642, -5.6199) centre (24.2675, -11.3478) ccw projected
  arc A311 (26.6642, -5.6199) -> (26.819, -4.8272) centre (0, 0) ccw projected
  arc A312 (26.819, -4.8272) -> (27.3555, -4.7983) centre (26.754, 1.3816) ccw projected
  arc A313 (27.3555, -4.7983) -> (28.1256, -4.6883) centre (26.5277, 3.7426) ccw projected
  arc A314 (28.1256, -4.6883) -> (29.1641, -4.4393) centre (26.0638, 6.2023) ccw projected
  arc A315 (29.1641, -4.4393) -> (29.2716, -3.6638) centre (0, 0) ccw projected
  arc A316 (29.2716, -3.6638) -> (28.3332, -3.1383) centre (23.3927, -13.0603) ccw projected
  arc A317 (28.3332, -3.1383) -> (27.629, -2.8262) centre (24.5084, -10.8197) ccw projected
  arc A318 (27.629, -2.8262) -> (27.1206, -2.6525) centre (25.3685, -8.6093) ccw projected
  arc A319 (27.1206, -2.6525) -> (27.1873, -1.8476) centre (0, 0) ccw projected
  arc A320 (27.1873, -1.8476) -> (27.7173, -1.7599) centre (26.4396, 4.3163) ccw projected
  arc A321 (27.7173, -1.7599) -> (28.4707, -1.5658) centre (25.955, 6.6382) ccw projected
  arc A322 (28.4707, -1.5658) -> (29.4754, -1.2041) centre (25.2233, 9.0318) ccw projected
  arc A323 (29.4754, -1.2041) -> (29.497, -0.4215) centre (0, 0) ccw projected
  arc A324 (29.497, -0.4215) -> (28.5065, -0.0023) centre (24.6875, -10.4076) ccw projected
  arc A325 (28.5065, -0.0023) -> (27.7722, 0.2303) centre (25.5499, -8.0579) ccw projected
  arc A326 (27.7722, 0.2303) -> (27.2478, 0.3471) centre (26.1617, -5.7663) ccw projected
  arc A327 (27.2478, 0.3471) -> (27.2255, 1.1544) centre (0, 0) ccw projected
  arc A328 (27.2255, 1.1544) -> (27.7427, 1.2999) centre (25.8043, 7.1987) ccw projected
  arc A329 (27.7427, 1.2999) -> (28.4701, 1.5757) centre (25.0672, 9.4531) ccw projected
  arc A330 (28.4701, 1.5757) -> (29.429, 2.0458) centre (24.0767, 11.7518) ccw projected
  arc A331 (29.429, 2.0458) -> (29.3643, 2.826) centre (0, 0) ccw projected
  arc A332 (29.3643, 2.826) -> (28.3412, 3.1318) centre (25.6826, -7.6286) ccw projected
  arc A333 (28.3412, 3.1318) -> (27.5783, 3.2841) centre (26.2813, -5.1983) ccw projected
  arc A334 (27.5783, 3.2841) -> (27.0442, 3.3425) centre (26.6372, -2.8533) ccw projected
  arc A335 (27.0442, 3.3425) -> (26.9333, 4.1425) centre (0, 0) ccw projected
  arc A336 (26.9333, 4.1425) -> (27.4313, 4.344) centre (24.8558, 9.9937) ccw projected
  arc A337 (27.4313, 4.344) -> (28.124, 4.6981) centre (23.8751, 12.1534) ccw projected
  arc A338 (28.124, 4.6981) -> (29.0253, 5.2708) centre (22.6377, 14.3291) ccw projected
  arc A339 (29.0253, 5.2708) -> (28.8752, 6.0392) centre (0, 0) ccw projected
  arc A340 (28.8752, 6.0392) -> (27.8246, 6.2305) centre (26.3659, -4.757) ccw projected
  arc A341 (27.8246, 6.2305) -> (27.0496, 6.298) centre (26.6936, -2.2756) ccw projected
  arc A342 (27.0496, 6.298) -> (26.5124, 6.2973) centre (26.7894, 0.0943) ccw projected
  arc A343 (26.5124, 6.2973) -> (26.3141, 7.0802) centre (0, 0) ccw projected
  arc A344 (26.3141, 7.0802) -> (26.787, 7.3353) centre (23.6055, 12.6674) ccw projected
  arc A345 (26.787, 7.3353) -> (27.4364, 7.7635) centre (22.3933, 14.7061) ccw projected
  arc A346 (27.4364, 7.7635) -> (28.2693, 8.4318) centre (20.924, 16.7325) ccw projected
  arc A347 (28.2693, 8.4318) -> (28.0356, 9.179) centre (0, 0) ccw projected
  arc A348 (28.0356, 9.179) -> (26.9703, 9.2537) centre (26.7292, -1.8277) ccw projected
  arc A349 (26.9703, 9.2537) -> (26.1926, 9.2355) centre (26.7819, 0.6748) ccw projected
  arc A350 (26.1926, 9.2355) -> (25.6587, 9.1756) centre (26.6165, 3.0408) ccw projected
  arc A351 (25.6587, 9.1756) -> (25.3755, 9.932) centre (0, 0) ccw projected
  arc A352 (25.3755, 9.932) -> (25.8175, 10.2375) centre (22.0687, 15.1873) ccw projected
  arc A353 (25.8175, 10.2375) -> (26.4159, 10.7346) centre (20.6396, 17.0802) ccw projected
  arc A354 (26.4159, 10.7346) -> (27.1702, 11.4905) centre (18.9563, 18.9327) ccw projected
  arc A355 (27.1702, 11.4905) -> (26.8557, 12.2075) centre (0, 0) ccw projected
  arc A356 (26.8557, 12.2075) -> (25.7887, 12.1645) centre (26.768, 1.1238) ccw projected
  arc A357 (25.7887, 12.1645) -> (25.0177, 12.0608) centre (26.5451, 3.6169) ccw projected
  arc A358 (25.0177, 12.0608) -> (24.4936, 11.9426) centre (26.1204, 5.9504) ccw projected
  arc A359 (24.4936, 11.9426) -> (24.1289, 12.6632) centre (0, 0) ccw projected
  arc A360 (24.1289, 12.6632) -> (24.5345, 13.0155) centre (20.2641, 17.5229) ccw projected
  arc A361 (24.5345, 13.0155) -> (25.0747, 13.5754) centre (18.6353, 19.2471) ccw projected
  arc A362 (25.0747, 13.5754) -> (25.7412, 14.4097) centre (16.7585, 20.9032) ccw projected
  arc A363 (25.7412, 14.4097) -> (25.3498, 15.0877) centre (0, 0) ccw projected
  arc A364 (25.3498, 15.0877) -> (24.294, 14.9276) centre (26.4819, 4.0617) ccw projected
  arc A365 (24.294, 14.9276) -> (23.5391, 14.7398) centre (25.9861, 6.5151) ccw projected
  arc A366 (23.5391, 14.7398) -> (23.0312, 14.5646) centre (25.3073, 8.7878) ccw projected
  arc A367 (23.0312, 14.5646) -> (22.5894, 15.2408) centre (0, 0) ccw projected
  arc A368 (22.5894, 15.2408) -> (22.9538, 15.6355) centre (18.2134, 19.6457) ccw projected
  arc A369 (22.9538, 15.6355) -> (23.4291, 16.2514) centre (16.4049, 21.1803) ccw projected
  arc A370 (23.4291, 16.2514) -> (23.9998, 17.154) centre (14.3573, 22.6199) ccw projected
  arc A371 (23.9998, 17.154) -> (23.5361, 17.7848) centre (0, 0) ccw projected
  arc A372 (23.5361, 17.7848) -> (22.5044, 17.5095) centre (25.8744, 6.9503) ccw projected
  arc A373 (22.5044, 17.5095) -> (21.7747, 17.2398) centre (25.1117, 9.3343) ccw projected
  arc A374 (21.7747, 17.2398) -> (21.2891, 17.0099) centre (24.187, 11.5184) ccw projected
  arc A375 (21.2891, 17.0099) -> (20.7757, 17.6333) centre (0, 0) ccw projected
  arc A376 (20.7757, 17.6333) -> (21.0945, 18.0658) centre (15.9417, 21.5301) ccw projected
  arc A377 (21.0945, 18.0658) -> (21.4991, 18.7302) centre (13.9753, 22.8564) ccw projected
  arc A378 (21.4991, 18.7302) -> (21.9671, 19.69) centre (11.7818, 24.062) ccw projected
  arc A379 (21.9671, 19.69) -> (21.4368, 20.2661) centre (0, 0) ccw projected
  arc A380 (21.4368, 20.2661) -> (20.4416, 19.8789) centre (24.9528, 9.7545) ccw projected
  arc A381 (20.4416, 19.8789) -> (19.746, 19.5306) centre (23.9325, 12.0401) ccw projected
  arc A382 (19.746, 19.5306) -> (19.2887, 19.2486) centre (22.773, 14.1093) ccw projected
  arc A383 (19.2887, 19.2486) -> (18.7098, 19.8118) centre (0, 0) ccw projected
  arc A384 (18.7098, 19.8118) -> (18.9791, 20.2767) centre (13.4764, 23.1532) ccw projected
  arc A385 (18.9791, 20.2767) -> (19.3081, 20.9816) centre (11.3761, 24.2551) ccw projected
  arc A386 (19.3081, 20.9816) -> (19.6677, 21.9871) centre (9.0632, 25.2121) ccw projected
  arc A387 (19.6677, 21.9871) -> (19.0773, 22.5013) centre (0, 0) ccw projected
  arc A388 (19.0773, 22.5013) -> (18.1307, 22.007) centre (23.7282, 12.4403) ccw projected
  arc A389 (18.1307, 22.007) -> (17.4777, 21.5843) centre (22.4627, 14.5998) ccw projected
  arc A390 (17.4777, 21.5843) -> (17.0541, 21.2537) centre (21.0827, 16.5289) ccw projected
  arc A391 (17.0541, 21.2537) -> (16.4168, 21.7498) centre (0, 0) ccw projected
  arc A392 (16.4168, 21.7498) -> (16.6333, 22.2415) centre (10.8476, 24.4952) ccw projected
  arc A393 (16.6333, 22.2415) -> (16.8828, 22.9783) centre (8.6388, 25.3594) ccw projected
  arc A394 (16.8828, 22.9783) -> (17.1295, 24.0173) centre (6.2347, 26.0561) ccw projected
  arc A395 (17.1295, 24.0173) -> (16.4862, 24.4634) centre (0, 0) ccw projected
  arc A396 (16.4862, 24.4634) -> (15.5997, 23.868) centre (22.2157, 14.9751) ccw projected
  arc A397 (15.5997, 23.868) -> (14.9971, 23.3759) centre (20.7203, 16.9823) ccw projected
  arc A398 (14.9971, 23.3759) -> (14.6125, 23.0008) centre (19.1364, 18.7478) ccw projected
  arc A399 (14.6125, 23.0008) -> (13.9245, 23.4237) centre (0, 0) ccw projected
  arc A400 (13.9245, 23.4237) -> (14.0856, 23.9363) centre (8.0871, 25.5398) ccw projected
  arc A401 (14.0856, 23.9363) -> (14.2525, 24.6961) centre (5.7966, 26.1558) ccw projected
  arc A402 (14.2525, 24.6961) -> (14.3835, 25.7559) centre (3.3305, 26.5838) ccw projected
  arc A403 (14.3835, 25.7559) -> (13.6949, 26.1285) centre (0, 0) ccw projected
  arc A404 (13.6949, 26.1285) -> (12.8793, 25.4392) centre (20.4335, 17.3281) ccw projected
  arc A405 (12.8793, 25.4392) -> (12.3346, 24.8839) centre (18.7263, 19.1586) ccw projected
  arc A406 (12.3346, 24.8839) -> (11.9936, 24.4687) centre (16.9579, 20.7392) ccw projected
  arc A407 (11.9936, 24.4687) -> (11.2632, 24.8134) centre (0, 0) ccw projected
  arc A408 (11.2632, 24.8134) -> (11.3669, 25.3405) centre (5.2284, 26.2744) ccw projected
  arc A409 (11.3669, 25.3405) -> (11.4492, 26.1141) centre (2.8841, 26.6347) ccw projected
  arc A410 (11.4492, 26.1141) -> (11.4628, 27.1819) centre (0.3858, 26.7888) ccw projected
  arc A411 (11.4628, 27.1819) -> (10.7375, 27.4765) centre (0, 0) ccw projected
  arc A412 (10.7375, 27.4765) -> (10.0026, 26.7016) centre (18.4032, 19.4708) ccw projected
  arc A413 (10.0026, 26.7016) -> (9.5223, 26.0897) centre (16.505, 21.1024) ccw projected
  arc A414 (9.5223, 26.0897) -> (9.229, 25.6396) centre (14.5734, 22.4788) ccw projected
  arc A415 (9.229, 25.6396) -> (8.4651, 25.9018) centre (0, 0) ccw projected
  arc A416 (8.4651, 25.9018) -> (8.5102, 26.4372) centre (2.3063, 26.6901) ccw projected
  arc A417 (8.5102, 26.4372) -> (8.507, 27.2151) centre (-0.0635, 26.7903) ccw projected
  arc A418 (8.507, 27.2151) -> (8.403, 28.2779) centre (-2.5635, 26.6687) ccw projected
  arc A419 (8.403, 28.2779) -> (7.6497, 28.4909) centre (0, 0) ccw projected
  arc A420 (7.6497, 28.4909) -> (7.0045, 27.6399) centre (16.1496, 21.3771) ccw projected
  arc A421 (7.0045, 27.6399) -> (6.5944, 26.9789) centre (14.0834, 22.79) ccw projected
  arc A422 (6.5944, 26.9789) -> (6.3525, 26.4992) centre (12.0121, 23.9456) ccw projected
  arc A423 (6.3525, 26.4992) -> (5.5644, 26.6758) centre (0, 0) ccw projected
  arc A424 (5.5644, 26.6758) -> (5.5503, 27.2129) centre (-0.6439, 26.7819) ccw projected
  arc A425 (5.5503, 27.2129) -> (5.4615, 27.9857) centre (-3.0102, 26.6208) ccw projected
  arc A426 (5.4615, 27.9857) -> (5.2412, 29.0307) centre (-5.4817, 26.2248) ccw projected
  arc A427 (5.2412, 29.0307) -> (4.469, 29.1595) centre (0, 0) ccw projected
  arc A428 (4.469, 29.1595) -> (3.9214, 28.2427) centre (13.6999, 23.024) ccw projected
  arc A429 (3.9214, 28.2427) -> (3.5865, 27.5406) centre (11.4909, 24.201) ccw projected
  arc A430 (3.5865, 27.5406) -> (3.3988, 27.0372) centre (9.305, 25.1217) ccw projected
  arc A431 (3.3988, 27.0372) -> (2.596, 27.1261) centre (0, 0) ccw projected
  arc A432 (2.596, 27.1261) -> (2.523, 27.6583) centre (-3.5862, 26.5485) ccw projected
  arc A433 (2.523, 27.6583) -> (2.3497, 28.4167) centre (-5.9205, 26.128) ccw projected
  arc A434 (2.3497, 28.4167) -> (2.0158, 29.431) centre (-8.3334, 25.4626) ccw projected
  arc A435 (2.0158, 29.431) -> (1.2341, 29.4742) centre (0, 0) ccw projected
  arc A436 (1.2341, 29.4742) -> (0.7907, 28.5027) centre (11.0839, 24.3913) ccw projected
  arc A437 (0.7907, 28.5027) -> (0.535, 27.768) centre (8.7588, 25.3182) ccw projected
  arc A438 (0.535, 27.768) -> (0.4038, 27.247) centre (6.485, 25.9929) ccw projected
  arc A439 (0.4038, 27.247) -> (-0.4038, 27.247) centre (0, 0) ccw projected
  arc A440 (-0.4038, 27.247) -> (-0.535, 27.768) centre (-6.485, 25.9929) ccw projected
  arc A441 (-0.535, 27.768) -> (-0.7907, 28.5027) centre (-8.7588, 25.3182) ccw projected
  arc A442 (-0.7907, 28.5027) -> (-1.2341, 29.4742) centre (-11.0839, 24.3913) ccw projected
  arc A443 (-1.2341, 29.4742) -> (-2.0158, 29.431) centre (0, 0) ccw projected
  arc A444 (-2.0158, 29.431) -> (-2.3517, 28.4093) centre (8.3334, 25.4626) ccw projected
  arc A445 (-2.3517, 28.4093) -> (-2.523, 27.6583) centre (5.9205, 26.128) ccw projected
  arc A446 (-2.523, 27.6583) -> (-2.596, 27.1261) centre (3.5862, 26.5485) ccw projected
  arc A447 (-2.596, 27.1261) -> (-3.3988, 27.0372) centre (0, 0) ccw projected
  arc A448 (-3.3988, 27.0372) -> (-3.5865, 27.5406) centre (-9.305, 25.1217) ccw projected
  arc A449 (-3.5865, 27.5406) -> (-3.9214, 28.2427) centre (-11.4909, 24.201) ccw projected
  arc A450 (-3.9214, 28.2427) -> (-4.469, 29.1595) centre (-13.6999, 23.024) ccw projected
  arc A451 (-4.469, 29.1595) -> (-5.2412, 29.0307) centre (0, 0) ccw projected
  arc A452 (-5.2412, 29.0307) -> (-5.4615, 27.9857) centre (5.4817, 26.2248) ccw projected
  arc A453 (-5.4615, 27.9857) -> (-5.5503, 27.2129) centre (3.0102, 26.6208) ccw projected
  arc A454 (-5.5503, 27.2129) -> (-5.5644, 26.6758) centre (0.6439, 26.7819) ccw projected
  arc A455 (-5.5644, 26.6758) -> (-6.3525, 26.4992) centre (0, 0) ccw projected
  arc A456 (-6.3525, 26.4992) -> (-6.5944, 26.9789) centre (-12.0121, 23.9456) ccw projected
  arc A457 (-6.5944, 26.9789) -> (-7.0045, 27.6399) centre (-14.0834, 22.79) ccw projected
  arc A458 (-7.0045, 27.6399) -> (-7.6497, 28.4909) centre (-16.1496, 21.3771) ccw projected
  arc A459 (-7.6497, 28.4909) -> (-8.403, 28.2779) centre (0, 0) ccw projected
  arc A460 (-8.403, 28.2779) -> (-8.507, 27.2151) centre (2.5635, 26.6687) ccw projected
  arc A461 (-8.507, 27.2151) -> (-8.5102, 26.4372) centre (0.0635, 26.7903) ccw projected
  arc A462 (-8.5102, 26.4372) -> (-8.4651, 25.9018) centre (-2.3063, 26.6901) ccw projected
  arc A463 (-8.4651, 25.9018) -> (-9.229, 25.6396) centre (0, 0) ccw projected
  arc A464 (-9.229, 25.6396) -> (-9.5223, 26.0897) centre (-14.5734, 22.4788) ccw projected
  arc A465 (-9.5223, 26.0897) -> (-10.0026, 26.7016) centre (-16.505, 21.1024) ccw projected
  arc A466 (-10.0026, 26.7016) -> (-10.7375, 27.4765) centre (-18.4032, 19.4708) ccw projected
  arc A467 (-10.7375, 27.4765) -> (-11.4628, 27.1819) centre (0, 0) ccw projected
  arc A468 (-11.4628, 27.1819) -> (-11.4492, 26.1141) centre (-0.3858, 26.7888) ccw projected
  arc A469 (-11.4492, 26.1141) -> (-11.3669, 25.3405) centre (-2.8841, 26.6347) ccw projected
  arc A470 (-11.3669, 25.3405) -> (-11.2632, 24.8134) centre (-5.2284, 26.2744) ccw projected
  arc A471 (-11.2632, 24.8134) -> (-11.9936, 24.4687) centre (0, 0) ccw projected
  arc A472 (-11.9936, 24.4687) -> (-12.3346, 24.8839) centre (-16.9579, 20.7392) ccw projected
  arc A473 (-12.3346, 24.8839) -> (-12.8793, 25.4392) centre (-18.7263, 19.1586) ccw projected
  arc A474 (-12.8793, 25.4392) -> (-13.6949, 26.1285) centre (-20.4335, 17.3281) ccw projected
  arc A475 (-13.6949, 26.1285) -> (-14.3835, 25.7559) centre (0, 0) ccw projected
  arc A476 (-14.3835, 25.7559) -> (-14.2525, 24.6961) centre (-3.3305, 26.5838) ccw projected
  arc A477 (-14.2525, 24.6961) -> (-14.0856, 23.9363) centre (-5.7966, 26.1558) ccw projected
  arc A478 (-14.0856, 23.9363) -> (-13.9245, 23.4237) centre (-8.0871, 25.5398) ccw projected
  arc A479 (-13.9245, 23.4237) -> (-14.6125, 23.0008) centre (0, 0) ccw projected
  arc A480 (6.2301, 4.7064) -> (5.9664, 4.5734) centre (6.6251, 3.5947) ccw projected
  arc A481 (7.3052, 4.9118) -> (6.2301, 4.7064) centre (7.3898, 1.5527) ccw projected
  arc A482 (10.1524, 4.3085) -> (7.3052, 4.9118) centre (7.4579, -1.3884) ccw projected
  arc A483 (10.2254, 4.1322) -> (10.1524, 4.3085) centre (0, 0) ccw projected
  arc A484 (8.6387, 1.6924) -> (10.2254, 4.1322) centre (4.2918, 6.2553) ccw projected
  arc A485 (7.7333, 1.0775) -> (8.6387, 1.6924) centre (6.3233, 4.1275) ccw projected
  arc A486 (7.4527, 0.985) -> (7.7333, 1.0775) centre (7.2265, 2.1428) ccw projected
  line L8 (6.5431, 0.8647) -> (7.4527, 0.985) projected
  arc A487 (6.5431, -0.8647) -> (6.5431, 0.8647) centre (0, 0) ccw projected
  line L9 (7.4527, -0.985) -> (6.5431, -0.8647) projected
  arc A488 (7.7333, -1.0775) -> (7.4527, -0.985) centre (7.2265, -2.1428) ccw projected
  arc A489 (8.6387, -1.6924) -> (7.7333, -1.0775) centre (6.3233, -4.1275) ccw projected
  arc A490 (10.2254, -4.1322) -> (8.6387, -1.6924) centre (4.2918, -6.2553) ccw projected
  arc A491 (10.1524, -4.3085) -> (10.2254, -4.1322) centre (0, 0) ccw projected
  arc A492 (7.3052, -4.9118) -> (10.1524, -4.3085) centre (7.4579, 1.3884) ccw projected
  arc A493 (6.2301, -4.7064) -> (7.3052, -4.9118) centre (7.3898, -1.5527) ccw projected
  arc A494 (5.9664, -4.5734) -> (6.2301, -4.7064) centre (6.6251, -3.5947) ccw projected
  line L10 (5.2381, -4.0152) -> (5.9664, -4.5734) projected
  arc A495 (4.0152, -5.2381) -> (5.2381, -4.0152) centre (0, 0) ccw projected
  line L11 (4.5734, -5.9664) -> (4.0152, -5.2381) projected
  arc A496 (4.7064, -6.2301) -> (4.5734, -5.9664) centre (3.5947, -6.6251) ccw projected
  arc A497 (4.9118, -7.3052) -> (4.7064, -6.2301) centre (1.5527, -7.3898) ccw projected
  arc A498 (4.3085, -10.1524) -> (4.9118, -7.3052) centre (-1.3884, -7.4579) ccw projected
  arc A499 (4.1322, -10.2254) -> (4.3085, -10.1524) centre (0, 0) ccw projected
  arc A500 (1.6924, -8.6387) -> (4.1322, -10.2254) centre (6.2553, -4.2918) ccw projected
  arc A501 (1.0775, -7.7333) -> (1.6924, -8.6387) centre (4.1275, -6.3233) ccw projected
  arc A502 (0.985, -7.4527) -> (1.0775, -7.7333) centre (2.1428, -7.2265) ccw projected
  line L12 (0.8647, -6.5431) -> (0.985, -7.4527) projected
  arc A503 (-0.8647, -6.5431) -> (0.8647, -6.5431) centre (0, 0) ccw projected
  line L13 (-0.985, -7.4527) -> (-0.8647, -6.5431) projected
  arc A504 (-1.0775, -7.7333) -> (-0.985, -7.4527) centre (-2.1428, -7.2265) ccw projected
  arc A505 (-1.6924, -8.6387) -> (-1.0775, -7.7333) centre (-4.1275, -6.3233) ccw projected
  arc A506 (-4.1322, -10.2254) -> (-1.6924, -8.6387) centre (-6.2553, -4.2918) ccw projected
  arc A507 (-4.3085, -10.1524) -> (-4.1322, -10.2254) centre (0, 0) ccw projected
  arc A508 (-4.9118, -7.3052) -> (-4.3085, -10.1524) centre (1.3884, -7.4579) ccw projected
  arc A509 (-4.7064, -6.2301) -> (-4.9118, -7.3052) centre (-1.5527, -7.3898) ccw projected
  arc A510 (-4.5734, -5.9664) -> (-4.7064, -6.2301) centre (-3.5947, -6.6251) ccw projected
  line L14 (-4.0152, -5.2381) -> (-4.5734, -5.9664) projected
  arc A511 (-5.2381, -4.0152) -> (-4.0152, -5.2381) centre (0, 0) ccw projected
  line L15 (-5.9664, -4.5734) -> (-5.2381, -4.0152) projected
  arc A512 (-6.2301, -4.7064) -> (-5.9664, -4.5734) centre (-6.6251, -3.5947) ccw projected
  arc A513 (-7.3052, -4.9118) -> (-6.2301, -4.7064) centre (-7.3898, -1.5527) ccw projected
  arc A514 (-10.1524, -4.3085) -> (-7.3052, -4.9118) centre (-7.4579, 1.3884) ccw projected
  arc A515 (-10.2254, -4.1322) -> (-10.1524, -4.3085) centre (0, 0) ccw projected
  arc A516 (-8.6387, -1.6924) -> (-10.2254, -4.1322) centre (-4.2918, -6.2553) ccw projected
  arc A517 (-7.7333, -1.0775) -> (-8.6387, -1.6924) centre (-6.3233, -4.1275) ccw projected
  arc A518 (-7.4527, -0.985) -> (-7.7333, -1.0775) centre (-7.2265, -2.1428) ccw projected
  line L16 (-6.5431, -0.8647) -> (-7.4527, -0.985) projected
  arc A519 (-6.5431, 0.8647) -> (-6.5431, -0.8647) centre (0, 0) ccw projected
  line L17 (-7.4527, 0.985) -> (-6.5431, 0.8647) projected
  arc A520 (-7.7333, 1.0775) -> (-7.4527, 0.985) centre (-7.2265, 2.1428) ccw projected
  arc A521 (-8.6387, 1.6924) -> (-7.7333, 1.0775) centre (-6.3233, 4.1275) ccw projected
  arc A522 (-10.2254, 4.1322) -> (-8.6387, 1.6924) centre (-4.2918, 6.2553) ccw projected
  arc A523 (-10.1524, 4.3085) -> (-10.2254, 4.1322) centre (0, 0) ccw projected
  arc A524 (-7.3052, 4.9118) -> (-10.1524, 4.3085) centre (-7.4579, -1.3884) ccw projected
  arc A525 (-6.2301, 4.7064) -> (-7.3052, 4.9118) centre (-7.3898, 1.5527) ccw projected
  arc A526 (-5.9664, 4.5734) -> (-6.2301, 4.7064) centre (-6.6251, 3.5947) ccw projected
  line L18 (-5.2381, 4.0152) -> (-5.9664, 4.5734) projected
  arc A527 (-4.0152, 5.2381) -> (-5.2381, 4.0152) centre (0, 0) ccw projected
  line L19 (-4.5734, 5.9664) -> (-4.0152, 5.2381) projected
  arc A528 (-4.7064, 6.2301) -> (-4.5734, 5.9664) centre (-3.5947, 6.6251) ccw projected
  arc A529 (-4.9118, 7.3052) -> (-4.7064, 6.2301) centre (-1.5527, 7.3898) ccw projected
  arc A530 (-4.3085, 10.1524) -> (-4.9118, 7.3052) centre (1.3884, 7.4579) ccw projected
  arc A531 (-4.1322, 10.2254) -> (-4.3085, 10.1524) centre (0, 0) ccw projected
  arc A532 (-1.6924, 8.6387) -> (-4.1322, 10.2254) centre (-6.2553, 4.2918) ccw projected
  arc A533 (-1.0775, 7.7333) -> (-1.6924, 8.6387) centre (-4.1275, 6.3233) ccw projected
  arc A534 (-0.985, 7.4527) -> (-1.0775, 7.7333) centre (-2.1428, 7.2265) ccw projected
  line L20 (-0.8647, 6.5431) -> (-0.985, 7.4527) projected
  arc A535 (0.8647, 6.5431) -> (-0.8647, 6.5431) centre (0, 0) ccw projected
  line L21 (0.985, 7.4527) -> (0.8647, 6.5431) projected
  arc A536 (1.0775, 7.7333) -> (0.985, 7.4527) centre (2.1428, 7.2265) ccw projected
  arc A537 (1.6924, 8.6387) -> (1.0775, 7.7333) centre (4.1275, 6.3233) ccw projected
  arc A538 (4.1322, 10.2254) -> (1.6924, 8.6387) centre (6.2553, 4.2918) ccw projected
  arc A539 (4.3085, 10.1524) -> (4.1322, 10.2254) centre (0, 0) ccw projected
  arc A540 (4.9118, 7.3052) -> (4.3085, 10.1524) centre (-1.3884, 7.4579) ccw projected
  arc A541 (4.7064, 6.2301) -> (4.9118, 7.3052) centre (1.5527, 7.3898) ccw projected
  arc A542 (4.5734, 5.9664) -> (4.7064, 6.2301) centre (3.5947, 6.6251) ccw projected
  line L22 (4.0152, 5.2381) -> (4.5734, 5.9664) projected
  arc A543 (5.2381, 4.0152) -> (4.0152, 5.2381) centre (0, 0) ccw projected
  line L23 (5.9664, 4.5734) -> (5.2381, 4.0152) projected
  circle A544 centre (0, 0) radius 2.995 projected
equation "\"d9\" = d10"
equation "\"d11\" = d9"
equation "\"d12\" = d11"
equation "\"d13\" = d12"
equation "\"d14\" = d13"
equation "\"d15\" = d13"
equation "\"d16\" = d15"
equation "\"d18\" = d17"
equation "\"d19\" = d18"
equation "\"d20\" = d19"
equation "\"d21\" = d20"
equation "\"d22\" = d21"
equation "\"d23\" = d17"
equation "\"d24\" = d23"
